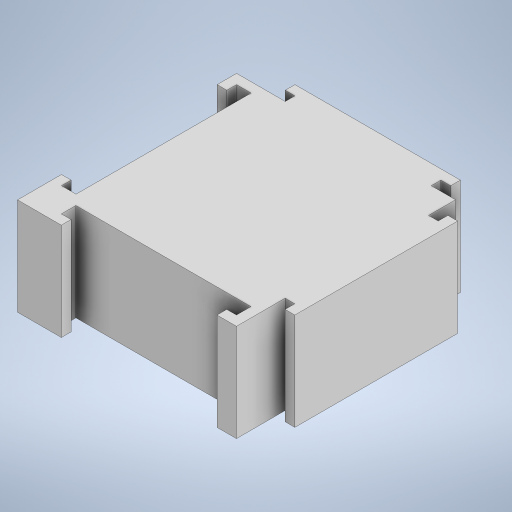
# Autodesk Inventor part: Maschio-femmina
Saved by Autodesk Inventor 2024 (Build 280153000, 153)
## iProperties
Created: 2024-01-14
Part Number: Maschio-femmina
Material: Generico
Document SubType Name: Modeling
Designer: Leonardo
Density: 1 g/cm^3
Appearance: Default
Author: Leonardo
Autodesk Inventor part; units mm, degrees
ref_plane "YZ Plane" through (0, 0, 0) normal (1, 0, 0) x (0, 1, 0)
ref_plane "XZ Plane" through (0, 0, 0) normal (0, 1, 0) x (-1, 0, 0)
ref_plane "XY Plane" through (0, 0, 0) normal (0, 0, 1) x (1, 0, 0)
sketch "Schizzo1" plane through (0, 0, 0) normal (0, 1, 0) x (-1, 0, 0)
  line L0 (10.0009, -10.0148) -> (9.0009, -10.0148)
  line L1 (-10, 9) -> (-10, 10)
  line L2 (11.5009, -9.0148) -> (10.0009, -9.0148)
  line L3 (10.0009, 8.9852) -> (10.0009, -9.0148)
  line L4 (-10, 12) -> (-10, 10)
  line L5 (9, 10) -> (-9, 10)
  line L6 (-10, -10.0148) -> (-9, -10.0148)
  line L7 (9.0009, -10.0148) -> (8.0009, -10.0148)
  line L8 (-9, -10.0148) -> (-8, -10.0148)
  line L9 (-10, 9) -> (-10, 8)
  line L10 (-10, -10.0148) -> (-10, -7.7324)
  circle A0 centre (-0.6701, -0.7825) radius 9.5
  line L11 (11.5009, -9.0148) -> (11.5009, -8.0148)
  line L12 (11.5009, -8.0148) -> (12.5009, -8.0148)
  line L13 (12.5009, -8.0148) -> (12.5009, -10.0148)
  line L14 (12.5009, -10.0148) -> (10.0009, -10.0148)
  line L15 (10.0009, 8.9852) -> (11.5009, 8.9852)
  line L16 (11.5009, 8.9852) -> (11.5009, 7.9852)
  line L17 (11.5009, 7.9852) -> (12.5009, 7.9852)
  line L18 (12.5009, 7.9852) -> (12.5009, 9.9852)
  line L19 (9, 10) -> (9, 11.5)
  line L20 (9, 11.5) -> (8, 11.5)
  line L21 (8, 11.5) -> (8, 12.5)
  line L22 (8, 12.5) -> (10, 12.5)
  line L23 (12.5009, 9.9852) -> (12.5009, 12.5)
  line L24 (12.5009, 12.5) -> (10, 12.5)
  line L25 (-9, 10) -> (-9, 11.5)
  line L26 (-9, 11.5) -> (-8, 11.5)
  line L27 (-8, 11.5) -> (-8, 12.5)
  line L28 (-8, 12.5) -> (-10, 12.5)
  line L29 (-10, 12.5) -> (-10, 12)
  line L30 (-10, -7.7324) -> (-10, -7.2324)
  line L31 (-10, -7.2324) -> (-11, -7.2324)
  line L32 (-11, -7.2324) -> (-11, -7.7324)
  line L33 (-11, -8.2324) -> (-12, -8.2324)
  line L34 (-11, -8.2324) -> (-11, -7.7324)
  line L35 (-10, 8) -> (-10, 7.5)
  line L36 (-10, 7.5) -> (-11, 7.5)
  line L37 (-11, 7.5) -> (-11, 8)
  line L38 (-11, 8.5) -> (-12, 8.5)
  line L39 (-11, 8) -> (-11, 8.5)
  line L40 (-12, -8.2324) -> (-12, 8.5)
  line L41 (8.0009, -10.0148) -> (7.5009, -10.0148)
  line L42 (7.5009, -10.0148) -> (7.5009, -11.0148)
  line L43 (7.5009, -11.0148) -> (8.5009, -11.0148)
  line L44 (8.5009, -11.0148) -> (8.5, -12.0148)
  line L45 (-8, -10.0148) -> (-7.5, -10.0148)
  line L46 (-7.5, -10.0148) -> (-7.5, -11.0148)
  line L47 (-7.5, -11.0148) -> (-8.5, -11.0148)
  line L48 (-8.5, -11.0148) -> (-8.5, -12.0148)
  line L49 (-8.5, -12.0148) -> (8.5, -12.0148)
  point P0 (0, 0)
  dimension "d24" = 1.5
  dimension "d36" = 1
  dimension "d43" = 1
  dimension "d44" = 1
  dimension "d45" = 2
  dimension "d46" = 1
  dimension "d47" = 1.5
  dimension "d48" = 1
  dimension "d49" = 1
  dimension "d51" = 1.5
  dimension "d53" = 1
  dimension "d54" = 2
  dimension "d55" = 0.5
  dimension "d56" = 0.5
  dimension "d58" = 1
  dimension "d59" = 0.5
  dimension "d60" = 1
  constraints: 100 end point, 21 perpendicular, 11 horizontal, 9 vertical, 1 centre point, 1 collinear
  measures "d24" distance of L2.start L2.end
  measures "d36" distance of L0.end L7.end
  measures "d43" distance of L2.start L11.end
  measures "d44" distance of L11.end L12.end
  measures "d45" distance of L12.end L13.end
  measures "d46" distance of L15.end L16.end
  measures "d47" distance of L5.start L19.end
  measures "d48" distance of L19.end L20.end
  measures "d49" distance of L20.end L21.end
  measures "d51" distance of L5.end L25.end
  measures "d53" distance of L25.end L26.end
  measures "d54" distance of L27.end L28.end
  measures "d55" distance of L10.end L30.end
  measures "d56" distance of L9.end L35.end
  measures "d58" distance of L42.end L43.end
  measures "d59" distance of L8.end L45.end
  measures "d60" distance of L47.end L48.end
extrude "Estrusione2" add sketch "Schizzo1" along normal blind 10 contours L0 L7 L41 L42 L43 L44 L49 L48 L47 L46 L45 L8 L6 L10 L30 L31 L32 L34 L33 L40 L38 L39 L37 L36 L35 L9 L1 L4 L29 L28 L27 L26 L25 L5 L19 L20 L21 L22 L24 L23 L18 L17 L16 L15 L3 L2 L11 L12 L13 L14 | A0
